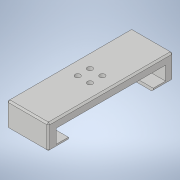
# Autodesk Inventor part: Grabber Platform
Saved by Autodesk Inventor 2022 (Build 260153000, 153)
## iProperties
Created: 2020-12-03
Part Number: Grabber Platform
Material: Generic
Document SubType Name: Modeling
Designer: caleb
Density: 1 g/cm^3
Appearance: Default
Author: caleb
Autodesk Inventor part; units mm, degrees
ref_plane "YZ Plane" through (0, 0, 0) normal (1, 0, 0) x (0, 1, 0)
ref_plane "XZ Plane" through (0, 0, 0) normal (0, 1, 0) x (-1, 0, 0)
ref_plane "XY Plane" through (0, 0, 0) normal (0, 0, 1) x (1, 0, 0)
sketch "Sketch1" plane through (0, 0, 0) normal (0, 1, 0) x (-1, 0, 0)
  line L0 (-13.5, 40.5) -> (13.5, 40.5)
  line L1 (13.5, 40.5) -> (13.5, -40.5)
  line L2 (13.5, -40.5) -> (-13.5, -40.5)
  line L3 (-13.5, -40.5) -> (-13.5, 40.5)
  line L4 (-13.5, 40.5) -> (13.5, -40.5) construction
  line L5 (13.5, 40.5) -> (-13.5, -40.5) construction
  point P0 (0, 0)
  dimension "d0" = 81
  dimension "d1" = 27
  constraints: 12 end point, 2 midpoint, 2 parallel, 1 horizontal, 1 perpendicular
  measures "d0" distance of L0.end L1.end
  measures "d1" distance of L0.start L0.end
extrude "Extrusion1" add sketch "Sketch1" along normal blind 16
sketch "Sketch4" plane through (13.5, 0, 40.5) normal (1, 0, 0) x (0, 0, -1)
  line L0 (13, 0) -> (13, 2)
  line L1 (13, 2) -> (5, 2)
  line L2 (5, 2) -> (5, 11)
  line L3 (5, 11) -> (76, 11)
  line L4 (76, 11) -> (76, 2)
  line L5 (76, 2) -> (68, 2)
  line L6 (68, 2) -> (68, 0)
  line L7 (0, 0) -> (81, 0) projected
  line L8 (0, 0) -> (0, 16) projected
  line L9 (81, 0) -> (81, 16) projected
  line L10 (81, 0) -> (0, 0) projected
  line L11 (0, 16) -> (81, 16) projected
  point P0 (40.5, 0)
  dimension "d28" = 2
  dimension "d29" = 8
  dimension "d32" = 8
  dimension "d33" = 5
  dimension "d35" = 2
  dimension "d39" = 5
  dimension "d40" = 5
  constraints: 14 end point, 5 perpendicular, 4 point on line, 1 vertical
  measures "d28" distance of L0.start L0.end
  measures "d29" distance of L0.end L1.end
  measures "d32" distance of L4.end L5.end
  measures "d33" distance between parallel lines of L8 L2
  measures "d35" distance of L5.end L6.end
  measures "d39" distance between parallel lines of L11 L3
  measures "d40" distance between parallel lines of L4 L9
extrude "Extrusion2" cut sketch "Sketch4" against normal through all contours L0 L1 L2 L3 L4 L5 L6 L7
sketch "Sketch2" plane through (0.35, 11, 3.15) normal (0, -1, 0) x (1, 0, 0)
  circle A0 centre (3.65, -7.15) radius 1.5
  circle A1 centre (3.65, 0.85) radius 1.5
  circle A2 centre (-4.35, 0.85) radius 1.5
  circle A3 centre (-4.35, -7.15) radius 1.5
  point P0 (-0.35, -3.15)
  dimension "d4" = 3
  dimension "d5" = 4
  dimension "d6" = 4
  dimension "d7" = 4
  dimension "d8" = 4
  constraints: 4 centre point, 3 equal radius, 2 horizontal alignment, 2 vertical alignment
  measures "d4" diameter of A1
  measures "d5" horizontal distance of point (-0.35, -3.15) A1.centre
  measures "d6" horizontal distance of A1.centre point (-0.35, -3.15)
  measures "d7" horizontal distance of point (-0.35, -3.15) A0.centre
  measures "d8" horizontal distance of point (-0.35, -3.15) A3.centre
hole "Hole1" at (4, 11, 4) at (4, 11, -4) at (-4, 11, -4) at (-4, 11, 4) direction (0, 1, 0) diameter 3.4 end through all countersink diameter 6.3 countersink angle 90 clearance for "Flat Head Machine Screw" size "M3" standard "Ansi Metric M Profile"
chamfer "Chamfer1" distance 1 angle 45 14 edges at (13.5, 16, 0) (13.5, 8, 40.5) (0, 0, 40.5) (0, 16, 40.5) (-13.5, 16, 0) (-13.5, 8, 40.5) (13.5, 0, 34) (13.5, 0, -34) (13.5, 8, -40.5) (0, 16, -40.5) (0, 0, -40.5) (-13.5, 8, -40.5) (-13.5, 0, -34) (-13.5, 0, 34)
body "Solid1"
